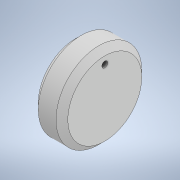
# Autodesk Inventor part: 711138 (Доделать)
Saved by Autodesk Inventor 2022 (Build 260153000, 153)
## iProperties
Created: 2021-10-22
Part Number: 711138 (Доделать)
Material: Типовые
Document SubType Name: Modeling
Designer: RaNSiD
Density: 1 g/cm^3
Appearance: По умолчанию
Author: RaNSiD
Autodesk Inventor part; units mm, degrees
ref_plane "YZ Plane" through (0, 0, 0) normal (1, 0, 0) x (0, 1, 0)
ref_plane "XZ Plane" through (0, 0, 0) normal (0, 1, 0) x (-1, 0, 0)
ref_plane "XY Plane" through (0, 0, 0) normal (0, 0, 1) x (1, 0, 0)
sketch "Эскиз5" plane through (0, 0, 0) normal (0, 0, 1) x (1, 0, 0)
  line L0 (0, 0) -> (20, 0)
  line L1 (20, 0) -> (20, 25)
  line L2 (16, 29) -> (4, 29)
  line L3 (0, 25) -> (0, 0)
  line L4 (4, 29) -> (0, 25)
  line L5 (16, 29) -> (20, 25)
  point P0 (20, 29)
  point P1 (0, 29)
  dimension "d42" = 20
  dimension "d43" = 29
  dimension "d44" = 4
  dimension "d45" = 4
  dimension "d46" = 4
  dimension "d47" = 4
  constraints: 12 end point, 4 point on line, 2 parallel, 1 horizontal, 1 perpendicular
  measures "d42" distance of point (0, 29) point (20, 29)
  measures "d43" distance of point (20, 29) L0.end
  measures "d44" distance of L2.end point (0, 29)
  measures "d45" distance of L3.start point (0, 29)
  measures "d46" distance of L2.start point (20, 29)
  measures "d47" distance of L1.end point (20, 29)
revolve "Вращение3" add sketch "Эскиз5" angle 360 about axis through (0, 0, 0) along (1, 0, 0)
sketch "Эскиз6" plane through (0, 0, 0) normal (-1, 0, 0) x (0, 0, 1)
  point P0 (0, 0)
  point P1 (0, 0)
  constraints: 1 coincident
hole "Отверстие3" at (0, 0, 0) direction (1, 0, 0) diameter 6 depth 8 tip angle 140 countersink diameter 7 countersink angle 90
sketch "Эскиз8" plane through (0, 0, 0) normal (-1, 0, 0) x (0, 0, 1)
  line L0 (0, 0) -> (0, 23) construction
  dimension "d56" = 23
  constraints: 2 end point, 1 coincident, 1 vertical
  measures "d56" distance of L0.start L0.end
hole "Отверстие4" at (0, 23, 0) direction (1, 0, 0) diameter 4 depth 4
sketch "Эскиз9" plane through (20, 0, 0) normal (1, 0, 0) x (0, 0, -1)
  line L0 (0, 0) -> (0, 20) construction
  dimension "d64" = 20
  constraints: 2 end point, 1 coincident, 1 vertical
  measures "d64" distance of L0.start L0.end
hole "Отверстие5" at (20, 20, 0) direction (-1, 0, 0) diameter 4 depth 4 tip angle 118
thread "Резьба3" size "M6x1" class "6H" standard "ANSI Metric M Profile" full length
equation "\"d45\" = d44"
equation "\"d46\" = d44"
equation "\"d47\" = d46"
